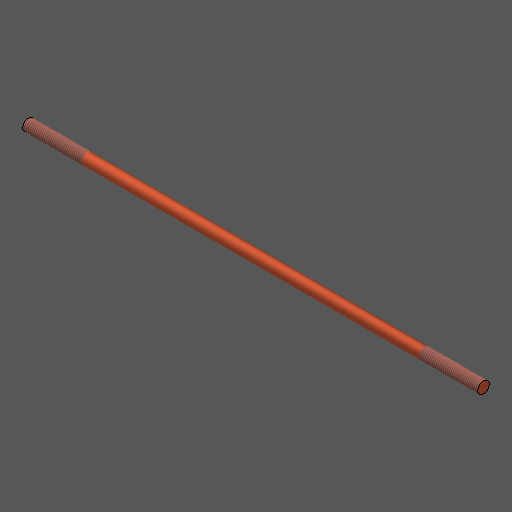
# Autodesk Inventor part: feed-rod
Saved by Autodesk Inventor 2025 (Build 290162000, 162)
## iProperties
Created: 2024-05-16
Part Number: feed-rod
Material: Copper
Document SubType Name: Modeling
Designer: AK
Density: 8.94 g/cm^3
Appearance: Copper - Satin
Mass: 27.4776 g
Surface Area: 24.216 cm^2
Volume: 3.4347 cm^3
Author: AK
Title: vacuum feed copper rod
Autodesk Inventor part; units mm, degrees
ref_plane "YZ Plane" through (0, 0, 0) normal (1, 0, 0) x (0, 1, 0)
ref_plane "XZ Plane" through (0, 0, 0) normal (0, 1, 0) x (-1, 0, 0)
ref_plane "XY Plane" through (0, 0, 0) normal (0, 0, 1) x (1, 0, 0)
sketch "sketch1" plane through (0, 0, 0) normal (1, 0, 0) x (0, 1, 0)
  circle A0 centre (0, 0) radius 2.5
  dimension "d0" = 5
  constraints: 1 centre point, 1 coincident
  measures "d0" diameter of A0
extrude "押し出し1" add sketch "sketch1" along normal blind 200
thread "Thread1" size "M5x0.8" class "6g" standard "ANSI Metric M Profile" length 26
thread "Thread2" size "M5x0.8" class "6g" standard "ANSI Metric M Profile" length 26
